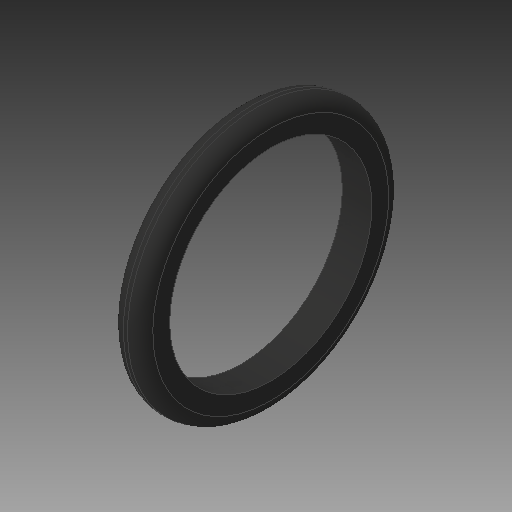
# Autodesk Inventor part: RuedaTrasera
Saved by Autodesk Inventor 2019.2 (Build 232265000, 265)
## iProperties
Created: 2017-04-06
Part Number: RuedaTrasera
Material: Rubber
Document SubType Name: Modeling
Designer: eroldan
Density: 0.93 g/cm^3
Appearance: Rubber - Black
Author: eroldan
Autodesk Inventor part; units mm, degrees
ref_plane "YZ Plane" through (0, 0, 0) normal (1, 0, 0) x (0, 1, 0)
ref_plane "XZ Plane" through (0, 0, 0) normal (0, 1, 0) x (-1, 0, 0)
ref_plane "XY Plane" through (0, 0, 0) normal (0, 0, 1) x (1, 0, 0)
sketch "Sketch5" plane through (0, 0, 0) normal (0, 0, 1) x (1, 0, 0)
  line L0 (-35, 310) -> (35, 310)
  line L1 (35, 310) -> (35, 240)
  line L2 (35, 240) -> (-35, 240)
  line L3 (-35, 240) -> (-35, 310)
  line L4 (-35, 310) -> (35, 240) construction
  line L5 (35, 310) -> (-35, 240) construction
  line L6 (-49, 0) -> (49, 0) projected
  point P0 (0, 0)
  point P1 (0, 310)
  point P2 (0, 275)
  point P3 (0, 310)
  dimension "d15" = 310
  dimension "d16" = 70
  dimension "d17" = 70
  constraints: 12 end point, 3 midpoint, 2 parallel, 1 coincident, 1 horizontal, 1 perpendicular
  measures "d15" distance of point (0, 0) point (0, 310)
  measures "d16" distance of L1.end L2.end
  measures "d17" distance of L0.end L1.end
revolve "Revolution3" add sketch "Sketch5" angle 360 about axis through (-10, 0, 0) along (1, 0, 0)
fillet "Fillet1" radius 30 2 edges at (35, -310, 0) (-35, -310, 0)
body "Solid1"
body "Solid3"
